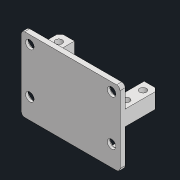
# Autodesk Inventor part: MotorCasingSmall
Saved by Autodesk Inventor 2022.2 (Build 262287010, 287A)
## iProperties
Created: 2022-06-04
Part Number: MotorCasingSmall
Material: Generic
Document SubType Name: Modeling
Designer: frede
Density: 1 g/cm^3
Appearance: Default
Author: frede
Autodesk Inventor part; units mm, degrees
ref_plane "YZ Plane" through (0, 0, 0) normal (1, 0, 0) x (0, 1, 0)
ref_plane "XZ Plane" through (0, 0, 0) normal (0, 1, 0) x (-1, 0, 0)
ref_plane "XY Plane" through (0, 0, 0) normal (0, 0, 1) x (1, 0, 0)
sketch "Sketch1" plane through (0, 0, 0) normal (0, 0, 1) x (1, 0, 0)
  line L0 (-29, 12.3) -> (29, 12.3)
  line L1 (29, 12.3) -> (29, -31.3)
  line L2 (29, -31.3) -> (-29, -31.3)
  line L3 (-29, -31.3) -> (-29, 12.3)
  line L4 (-15.4526, -28.3) -> (15.4526, -28.3) construction
  line L5 (-27, 2.4) -> (-27, 0) construction
  line L6 (15.475, 12.3) -> (4.725, 12.3) construction
  point P0 (0, 12.3)
  point P1 (0, -31.3)
  point P2 (0, 0)
  point P3 (10.1, 12.3)
  dimension "MotorMountBaseBracketOffset" = 2
  dimension "MotorMountBaseBottomOffset" = 3
  constraints: 8 end point, 3 midpoint, 2 parallel, 1 horizontal, 1 perpendicular, 1 point on line, 1 vertical alignment
  measures "MotorMountBaseBracketOffset" distance between parallel lines of L3 L5
  measures "MotorMountBaseBottomOffset" distance between parallel lines of L2 L4
extrude "Extrusion1" add sketch "Sketch1" along normal blind 3
sketch "Sketch2" plane through (0, 0, 0) normal (0, 0, -1) x (-1, 0, 0)
  line L0 (-29, -31.3) -> (-29, 12.3) construction
  line L1 (-26, 0) -> (-19.25, 0) construction
  line L2 (-19.95, -21.3) -> (-19.95, -0.5) construction
  line L3 (-29, -9.5) -> (-20.45, -9.5)
  line L4 (-20.45, -9.5) -> (-20.45, -0.5)
  line L5 (-20.45, -0.5) -> (-29, -0.5)
  line L6 (-29, -0.5) -> (-29, -9.5)
  dimension "d66" = 9
  dimension "d67" = 0.5
  dimension "d68" = 0.5
  constraints: 8 end point, 2 parallel, 1 horizontal, 1 midpoint, 1 perpendicular
  measures "d66" distance of L5.end L3.start
  measures "d67" distance between parallel lines of L1 L5
  measures "d68" distance between parallel lines of L2 L4
extrude "Extrusion6" add sketch "Sketch2" along normal blind 19.7
sketch "Sketch7" plane through (0, 0, 0) normal (0, 0, -1) x (-1, 0, 0)
  line L0 (-16.8094, -28.4) -> (-16.8094, -30.4)
  line L1 (-18.8094, -28.4) -> (-16.8094, -28.4)
  line L2 (-20.05, -26.1255) -> (-18.8094, -28.4)
  line L3 (-20.05, -24.1255) -> (-20.05, -26.1255)
  line L4 (-22.05, -24.1255) -> (-20.05, -24.1255)
  line L5 (-22.05, -30.4) -> (-22.05, -24.1255)
  line L6 (-16.8094, -30.4) -> (-22.05, -30.4)
  line L7 (15.4526, -28.3) -> (-15.4526, -28.3) construction
  line L8 (-19.35, -27.2) -> (-18.75, -28.3) construction
  line L9 (-19.95, -21.3) -> (-19.95, -0.5) construction
  point P0 (0, 0)
  dimension "d79" = 2
  dimension "d82" = 0.1
  dimension "d83" = 0.1
  dimension "d84" = 0.1
  constraints: 14 end point, 5 perpendicular, 2 vertical, 1 horizontal, 1 parallel
  measures "d79" distance of L0.start L0.end
  measures "d82" distance between parallel lines of L9 L3
  measures "d83" distance between parallel lines of L8 L2
  measures "d84" distance between parallel lines of L7 L1
extrude "Extrusion7" add sketch "Sketch7" along normal blind 4
sketch "Sketch5" plane through (0, 0, 0) normal (0, 0, -1) x (-1, 0, 0)
  circle A0 centre (-24, 7.3) radius 2.5
  circle A1 centre (-24, -19.3) radius 2.5
  point P0 (0, 0)
  point P1 (-29, -31.3)
  point P2 (-29, 12.3)
  dimension "d89" = 5
  dimension "d90" = 5
  dimension "d91" = 5
  dimension "MotorMountBottomHoleOffset" = 12
  constraints: 2 centre point, 1 equal radius, 1 vertical alignment
  measures "d89" diameter of A0
  measures "d90" horizontal distance of A0.centre point (-29, 12.3)
  measures "d91" horizontal distance of A0.centre point (-29, 12.3)
  measures "MotorMountBottomHoleOffset" vertical distance of A1.centre point (-29, -31.3)
extrude "Extrusion4" cut sketch "Sketch5" against normal through all
chamfer "Chamfer1" distance 1.5 angle 45 2 edges at (26.5, 7.3, 0) (26.5, -19.3, 0)
chamfer "Chamfer4" distance 2 angle 45 2 edges at (29, -5, -19.7) (22.05, -30.4, -2)
sketch "Sketch8" plane through (20.45, -0.5, 0) normal (0, 1, 0) x (1, 0, 0)
  arc A0 (5.9164, 6.2173) -> (5.9164, 3.6327) centre (4.2611, 4.925) ccw construction
  arc A1 (5.9164, 16.0673) -> (5.9164, 13.4827) centre (4.2611, 14.775) ccw construction
  circle A2 centre (4.2611, 14.775) radius 2
  circle A3 centre (4.2611, 4.925) radius 2
  point P0 (-20.45, 0)
  dimension "MotorMountPillarHoleDia" = 4
  dimension "d99" = 4
  constraints: 2 centre point, 2 coincident
  measures "MotorMountPillarHoleDia" diameter of A2
  measures "d99" diameter of A3
extrude "Extrusion8" cut sketch "Sketch8" against normal through all
mirror "Mirror1" about plane through (0, 0, 0) normal (1, 0, 0) of "Extrusion7", "Extrusion4", "Chamfer1", "Extrusion6", "Chamfer4", "Extrusion8"
fillet "Fillet1" radius 2 4 edges at (29, -31.3, 1.5) (29, 12.3, 1.5) (-29, 12.3, 1.5) (-29, -31.3, 1.5)
equation "\"d66\" = MotorMountPillarDepth"
equation "\"d67\" = MotorMountPillarOffset"
equation "\"d68\" = MotorMountPillarOffset"
equation "\"d82\" = MotorMountLocatorOffset"
equation "\"d83\" = MotorMountLocatorOffset"
equation "\"d84\" = MotorMountLocatorOffset"
equation "\"d89\" = ScrewHoleDia"
equation "\"d90\" = 0.5 * ScrewPlateSize"
equation "\"d91\" = d90"
equation "\"d42\" = ScrewHoleFillet"
equation "\"d99\" = MotorMountPillarHoleDia"
equation "\"MotorMountPillarDepth\" = 9"
equation "\"MotorMountPillarOffset\" = 0.5"
equation "\"MotorMountLocatorOffset\" = 0.1"
equation "\"ScrewHoleDia\" = 5"
equation "\"ScrewHoleFillet\" = 1.5"
equation "\"ScrewPlateSize\" = 10"
body "Solid1"
